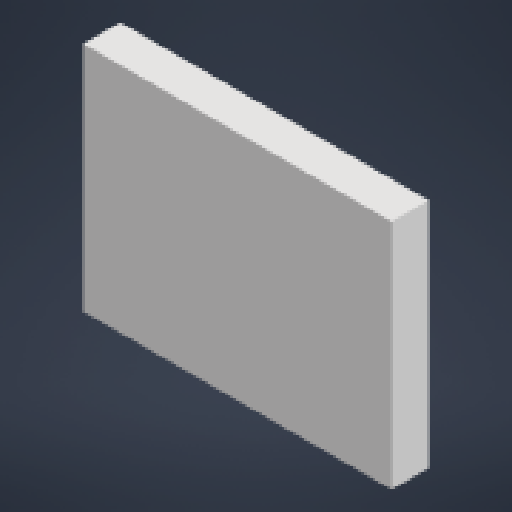
# Autodesk Inventor part: Part3
Saved by Autodesk Inventor 2025.2 (Build 292293000, 293)
## iProperties
Created: 2025-03-05
Part Number: Part3
Material: Generic
Document SubType Name: Modeling
Designer: cbast
Density: 1 g/cm^3
Appearance: Default
Author: cbast
Autodesk Inventor part; units mm, degrees
ref_plane "YZ Plane" through (0, 0, 0) normal (1, 0, 0) x (0, 1, 0)
ref_plane "XZ Plane" through (0, 0, 0) normal (0, 1, 0) x (-1, 0, 0)
ref_plane "XY Plane" through (0, 0, 0) normal (0, 0, 1) x (1, 0, 0)
sketch "Sketch1" plane through (0, 0, 0) normal (0, 0, 1) x (1, 0, 0)
  line L0 (-54, -57.15) -> (54, -57.15) construction
  line L1 (54, -57.15) -> (54, 57.15) construction
  line L2 (54, 57.15) -> (-54, 57.15) construction
  line L3 (-54, 57.15) -> (-54, -57.15) construction
  line L4 (-54, -57.15) -> (54, -57.15) construction
  line L5 (54, -57.15) -> (54, 57.15) construction
  line L6 (54, 57.15) -> (-54, 57.15) construction
  line L7 (-54, 57.15) -> (-54, -57.15) construction
  circle A0 centre (-9.5, -0.55) radius 9.5 construction
  circle A1 centre (10.5, -0.55) radius 9.5 construction
  line L8 (0, -0.55) -> (1, -0.55) construction
  line L9 (77.2, 10.9497) -> (83.8464, 10.9497) projected
  line L10 (83.8464, 10.9497) -> (83.8464, 62.15) projected
  line L11 (83.8464, 62.15) -> (-82.8464, 62.15) projected
  line L12 (-82.8464, 62.15) -> (-82.8464, 10.9497) projected
  line L13 (-82.8464, 10.9497) -> (-76.2, 10.9497) projected
  line L14 (-76.2, 10.9497) -> (-76.2, 57.15) projected
  line L15 (-76.2, 57.15) -> (77.2, 57.15) projected
  line L16 (77.2, 57.15) -> (77.2, 10.9497) projected
  circle A2 centre (20.5, 16.7705) radius 9.5 projected
  circle A3 centre (0.5, 16.7705) radius 9.5 projected
  line L17 (77.2, 10.9497) -> (77.2, 57.15) projected
  line L18 (77.2, 57.15) -> (-76.2, 57.15) projected
  line L19 (-76.2, 57.15) -> (-76.2, 10.9497) projected
  line L20 (-76.2, 10.9497) -> (-82.8464, 10.9497) projected
  line L21 (-82.8464, -12.0497) -> (-82.8464, 10.9497) projected
  line L22 (-76.2, -12.0497) -> (-82.8464, -12.0497) projected
  line L23 (-76.2, -12.0497) -> (-76.2, -58.25) projected
  line L24 (-76.2, -58.25) -> (77.2, -58.25) projected
  line L25 (77.2, -58.25) -> (77.2, -12.0497) projected
  line L26 (83.8464, -12.0497) -> (77.2, -12.0497) projected
  line L27 (83.8464, 10.9497) -> (83.8464, -12.0497) projected
  line L28 (83.8464, 10.9497) -> (77.2, 10.9497) projected
  circle A4 centre (-19.5, -17.8705) radius 9.5 projected
  circle A5 centre (-68.972, -26.5) radius 3.615 projected
  circle A6 centre (69.972, -26.5) radius 3.615 projected
  circle A7 centre (30.5, -0.55) radius 9.5 projected
  circle A8 centre (-29.5, -0.55) radius 9.5 projected
  circle A9 centre (10.5, -0.55) radius 9.5 projected
  circle A10 centre (-9.5, -0.55) radius 9.5 projected
  circle A11 centre (0.5, -17.8705) radius 9.5 projected
  circle A12 centre (20.5, -17.8705) radius 9.5 projected
  circle A13 centre (-68.972, 25.4) radius 3.615 projected
  circle A14 centre (69.972, 25.4) radius 3.615 projected
  circle A15 centre (-19.5, 16.7705) radius 9.5 projected
  line L29 (77.2, -12.0497) -> (77.2, -58.25) projected
  line L30 (83.8464, -12.0497) -> (77.2, -12.0497) projected
  line L31 (77.2, -12.0497) -> (77.2, -58.25) projected
  line L32 (77.2, -58.25) -> (-76.2, -58.25) projected
  line L33 (-76.2, -58.25) -> (-76.2, -12.0497) projected
  line L34 (-76.2, -12.0497) -> (-82.8464, -12.0497) projected
  line L35 (-82.8464, -12.0497) -> (-82.8464, -63.25) projected
  line L36 (-82.8464, -63.25) -> (83.8464, -63.25) projected
  line L37 (83.8464, -63.25) -> (83.8464, -12.0497) projected
  line L38 (83.8484, 61.7431) -> (83.8484, -63.6569) projected
  line L39 (83.8484, -63.6569) -> (103.8484, -63.6569) projected
  line L40 (103.8484, 61.7431) -> (103.8484, -63.6569) projected
  line L41 (83.8484, 61.7431) -> (103.8484, 61.7431) projected
  line L42 (-102.8465, 60.8533) -> (-102.8465, -64.5467) projected
  line L43 (-102.8465, 60.8533) -> (-102.8465, -64.5467) projected
  line L44 (-102.8465, -64.5467) -> (-82.8465, -64.5467) projected
  line L45 (-82.8465, 60.8533) -> (-82.8465, -64.5467) projected
  line L46 (-102.8465, 60.8533) -> (-82.8465, 60.8533) projected
  line L47 (-82.8464, -63.25) -> (83.8464, -63.25)
  line L48 (83.8464, -63.25) -> (83.8464, 62.15)
  line L49 (83.8464, 62.15) -> (-82.8464, 62.15)
  line L50 (-82.8464, 62.15) -> (-82.8464, -63.25)
  line L51 (-82.8464, -63.25) -> (83.8464, 62.15) construction
  line L52 (83.8464, -63.25) -> (-82.8464, 62.15) construction
  point P0 (0, 0)
  point P1 (0.5, -0.55)
  constraints: 14 end point, 4 horizontal alignment, 3 midpoint, 2 horizontal, 2 parallel, 1 perpendicular, 2 other
extrude "Extrusion1" add sketch "Sketch1" along normal blind 20 contours L16 L15 L14 L13 L12 L11 L10 L9 | L9 L27 L26 L25 L24 L23 L22 L21 L13 L14 L15 L16 | L37 L36 L35 L22 L23 L24 L25 L26 | A2 | A3 | A4 | A5 | A6 | A7 | A8 | A9 | A10 | A11 | A12 | A13 | A14 | A15
body "Solid1"
